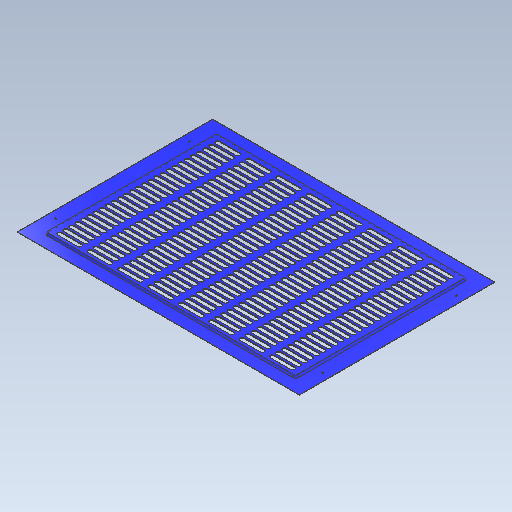
# Autodesk Inventor part: tapa_caja_calor
Saved by Autodesk Inventor 2021 (Build 250183000, 183)
## iProperties
Created: 2021-04-15
Part Number: tapa_caja_calor
Material: Acero AISI 1006 85 LC
Document SubType Name: Chapa
Designer: Leonardo Fabio Mercado Benítez
Density: 7.872 g/cm^3
Sheet Metal Rule: Por defecto_mm
Appearance: Acero
Mass: 732.482 g
Surface Area: 2149.19 cm^2
Volume: 93.049 cm^3
Flat Pattern Width: 32.15 cm
Flat Pattern Length: 46.42 cm
Flat Pattern Area: 1492.4 cm^2
Sheet Metal Width: 321,500 mm
Sheet Metal Length: 464,200 mm
Sheet Metal Area: 149240,300 mm^2
Author: Leonardo Fabio Mercado Benítez
Autodesk Inventor part; units mm, degrees
(part 1 of 3)
ref_plane "YZ Plane" through (0, 0, 0) normal (1, 0, 0) x (0, 1, 0)
ref_plane "XZ Plane" through (0, 0, 0) normal (0, 1, 0) x (-1, 0, 0)
ref_plane "XY Plane" through (0, 0, 0) normal (0, 0, 1) x (1, 0, 0)
sketch "Boceto1" plane through (0, 0, 0) normal (0, 1, 0) x (-1, 0, 0)
  line L0 (232.1, 160.75) -> (-232.1, 160.75)
  line L1 (-232.1, 160.75) -> (-232.1, -160.75)
  line L2 (-232.1, -160.75) -> (232.1, -160.75)
  line L3 (232.1, -160.75) -> (232.1, 160.75)
  line L4 (232.1, 160.75) -> (-232.1, -160.75) construction
  line L5 (-232.1, 160.75) -> (232.1, -160.75) construction
  point P0 (0, 0)
  dimension "d0" = 464.2
  dimension "d1" = 321.5
  measures "d0" distance of L2.end L1.end
  measures "d1" distance of L1.end L0.end
extrude "Placa1" add sketch "Boceto1" along normal blind 0.45
sketch "Boceto3" plane through (0, 0.45, 0) normal (0, 1, 0) x (1, 0, 0)
  line L0 (-201.7, -141.7) -> (201.7, -141.7)
  line L1 (206.7, -136.7) -> (206.7, 136.7)
  line L2 (201.7, 141.7) -> (-201.7, 141.7)
  line L3 (-206.7, 136.7) -> (-206.7, -136.7)
  line L4 (-206.7, -141.7) -> (206.7, 141.7) construction
  line L5 (206.7, -141.7) -> (-206.7, 141.7) construction
  arc A0 (-201.7, 141.7) -> (-206.7, 136.7) centre (-201.7, 136.7) ccw
  arc A1 (206.7, 136.7) -> (201.7, 141.7) centre (201.7, 136.7) ccw
  arc A2 (201.7, -141.7) -> (206.7, -136.7) centre (201.7, -136.7) ccw
  arc A3 (-206.7, -136.7) -> (-201.7, -141.7) centre (-201.7, -136.7) ccw
  line L6 (-201.7, 140.94) -> (201.7, 140.94)
  arc A4 (205.94, 136.7) -> (201.7, 140.94) centre (201.7, 136.7) ccw
  line L7 (205.94, 136.7) -> (205.94, -136.7)
  arc A5 (201.7, -140.94) -> (205.94, -136.7) centre (201.7, -136.7) ccw
  line L8 (201.7, -140.94) -> (-201.7, -140.94)
  arc A6 (-205.94, -136.7) -> (-201.7, -140.94) centre (-201.7, -136.7) ccw
  line L9 (-205.94, -136.7) -> (-205.94, 136.7)
  arc A7 (-201.7, 140.94) -> (-205.94, 136.7) centre (-201.7, 136.7) ccw
  point P0 (0, 0)
  dimension "d3" = 413.4
  dimension "d4" = 283.4
  dimension "d5" = 5
  dimension "d6" = 5
  dimension "d7" = 0.76
  constraints: 20 end point, 16 point on circle, 8 centre point, 8 point on line, 8 tangent, 4 parallel, 2 equal radius, 2 midpoint, 2 perpendicular, 1 horizontal, 7 other
  measures "d3" distance of L5.end L4.end
  measures "d4" distance of L4.end L5.start
  measures "d5" radius of A0
  measures "d6" radius of A1
  measures "d7" distance between parallel lines of L2 L6
sketch "Boceto3 outline for Extrusión1" plane through (0, 0.45, 0) normal (0, 1, 0) x (1, 0, 0)
  line L0 (-201.7, -141.7) -> (201.7, -141.7)
  arc A0 (-206.7, -136.7) -> (-201.7, -141.7) centre (-201.7, -136.7) ccw
  line L1 (-206.7, 136.7) -> (-206.7, -136.7)
  arc A1 (-201.7, 141.7) -> (-206.7, 136.7) centre (-201.7, 136.7) ccw
  line L2 (201.7, 141.7) -> (-201.7, 141.7)
  arc A2 (206.7, 136.7) -> (201.7, 141.7) centre (201.7, 136.7) ccw
  line L3 (206.7, -136.7) -> (206.7, 136.7)
  arc A3 (201.7, -141.7) -> (206.7, -136.7) centre (201.7, -136.7) ccw
extrude "Extrusión1" add sketch "Boceto3 outline for Extrusión1" along normal blind 3.175 draft -30
sketch "Boceto4" plane through (0, 0, 0) normal (0, -1, 0) x (1, 0, 0)
  line L0 (204.866913, -136.7) -> (204.866913, 136.7)
  line L1 (201.7, 139.866913) -> (-201.7, 139.866913)
  arc A0 (204.866913, 136.7) -> (201.7, 139.866913) centre (201.7, 136.7) ccw
  arc A1 (201.7, -139.866913) -> (204.866913, -136.7) centre (201.7, -136.7) ccw
  line L2 (-201.7, -139.866913) -> (201.7, -139.866913)
  arc A2 (-201.7, 139.866913) -> (-204.866913, 136.7) centre (-201.7, 136.7) ccw
  line L3 (-204.866913, 136.7) -> (-204.866913, -136.7)
  arc A3 (-204.866913, -136.7) -> (-201.7, -139.866913) centre (-201.7, -136.7) ccw
  point P0 (0, 0)
extrude "Extrusión2" cut sketch "Boceto4" against normal blind 2.415 draft -30
sketch "Boceto6" plane through (0, 2.415, 0) normal (0, -1, 0) x (1, 0, 0)
  line L0 (-194.972612, 131.472612) -> (-154.972612, 131.472612) construction
  line L1 (-191.622612, 128.122612) -> (-158.322612, 128.122612)
  line L2 (-158.322612, 134.822612) -> (-191.622612, 134.822612)
  arc A0 (-191.622612, 134.822612) -> (-191.622612, 128.122612) centre (-191.622612, 131.472612) ccw
  arc A1 (-158.322612, 128.122612) -> (-158.322612, 134.822612) centre (-158.322612, 131.472612) ccw
  line L3 (-203.472612, 136.7) -> (-203.472612, -136.7)
  line L4 (201.7, 138.472612) -> (-201.7, 138.472612)
  line L5 (-144.972612, 131.472612) -> (-104.972612, 131.472612) construction
  line L6 (-141.622612, 128.122612) -> (-108.322612, 128.122612)
  line L7 (-108.322612, 134.822612) -> (-141.622612, 134.822612)
  arc A2 (-141.622612, 134.822612) -> (-141.622612, 128.122612) centre (-141.622612, 131.472612) ccw
  arc A3 (-108.322612, 128.122612) -> (-108.322612, 134.822612) centre (-108.322612, 131.472612) ccw
  line L8 (-94.972612, 131.472612) -> (-54.972612, 131.472612) construction
  line L9 (-91.622612, 128.122612) -> (-58.322612, 128.122612)
  line L10 (-58.322612, 134.822612) -> (-91.622612, 134.822612)
  arc A4 (-91.622612, 134.822612) -> (-91.622612, 128.122612) centre (-91.622612, 131.472612) ccw
  arc A5 (-58.322612, 128.122612) -> (-58.322612, 134.822612) centre (-58.322612, 131.472612) ccw
  line L11 (-44.972612, 131.472612) -> (-4.972612, 131.472612) construction
  line L12 (-41.622612, 128.122612) -> (-8.322612, 128.122612)
  line L13 (-8.322612, 134.822612) -> (-41.622612, 134.822612)
  arc A6 (-41.622612, 134.822612) -> (-41.622612, 128.122612) centre (-41.622612, 131.472612) ccw
  arc A7 (-8.322612, 128.122612) -> (-8.322612, 134.822612) centre (-8.322612, 131.472612) ccw
  line L14 (5.027388, 131.472612) -> (45.027388, 131.472612) construction
  line L15 (8.377388, 128.122612) -> (41.677388, 128.122612)
  line L16 (41.677388, 134.822612) -> (8.377388, 134.822612)
  arc A8 (8.377388, 134.822612) -> (8.377388, 128.122612) centre (8.377388, 131.472612) ccw
  arc A9 (41.677388, 128.122612) -> (41.677388, 134.822612) centre (41.677388, 131.472612) ccw
  line L17 (55.027388, 131.472612) -> (95.027388, 131.472612) construction
  line L18 (58.377388, 128.122612) -> (91.677388, 128.122612)
  line L19 (91.677388, 134.822612) -> (58.377388, 134.822612)
  arc A10 (58.377388, 134.822612) -> (58.377388, 128.122612) centre (58.377388, 131.472612) ccw
  arc A11 (91.677388, 128.122612) -> (91.677388, 134.822612) centre (91.677388, 131.472612) ccw
  line L20 (105.027388, 131.472612) -> (145.027388, 131.472612) construction
  line L21 (108.377388, 128.122612) -> (141.677388, 128.122612)
  line L22 (141.677388, 134.822612) -> (108.377388, 134.822612)
  arc A12 (108.377388, 134.822612) -> (108.377388, 128.122612) centre (108.377388, 131.472612) ccw
  arc A13 (141.677388, 128.122612) -> (141.677388, 134.822612) centre (141.677388, 131.472612) ccw
  line L23 (155.027388, 131.472612) -> (195.027388, 131.472612) construction
  line L24 (158.377388, 128.122612) -> (191.677388, 128.122612)
  line L25 (191.677388, 134.822612) -> (158.377388, 134.822612)
  arc A14 (158.377388, 134.822612) -> (158.377388, 128.122612) centre (158.377388, 131.472612) ccw
  arc A15 (191.677388, 128.122612) -> (191.677388, 134.822612) centre (191.677388, 131.472612) ccw
  arc A16 (-158.322612, 118.122612) -> (-158.322612, 124.822612) centre (-158.322612, 121.472612) ccw
  line L26 (-191.622612, 118.122612) -> (-158.322612, 118.122612)
  line L27 (-158.322612, 124.822612) -> (-191.622612, 124.822612)
  arc A17 (-191.622612, 124.822612) -> (-191.622612, 118.122612) centre (-191.622612, 121.472612) ccw
  line L28 (-194.972612, 121.472612) -> (-154.972612, 121.472612) construction
  arc A18 (-158.322612, 108.122612) -> (-158.322612, 114.822612) centre (-158.322612, 111.472612) ccw
  line L29 (-191.622612, 108.122612) -> (-158.322612, 108.122612)
  line L30 (-158.322612, 114.822612) -> (-191.622612, 114.822612)
  arc A19 (-191.622612, 114.822612) -> (-191.622612, 108.122612) centre (-191.622612, 111.472612) ccw
  line L31 (-194.972612, 111.472612) -> (-154.972612, 111.472612) construction
  arc A20 (-158.322612, 98.122612) -> (-158.322612, 104.822612) centre (-158.322612, 101.472612) ccw
  line L32 (-191.622612, 98.122612) -> (-158.322612, 98.122612)
  line L33 (-158.322612, 104.822612) -> (-191.622612, 104.822612)
  arc A21 (-191.622612, 104.822612) -> (-191.622612, 98.122612) centre (-191.622612, 101.472612) ccw
  line L34 (-194.972612, 101.472612) -> (-154.972612, 101.472612) construction
  arc A22 (-158.322612, 88.122612) -> (-158.322612, 94.822612) centre (-158.322612, 91.472612) ccw
  line L35 (-191.622612, 88.122612) -> (-158.322612, 88.122612)
  line L36 (-158.322612, 94.822612) -> (-191.622612, 94.822612)
  arc A23 (-191.622612, 94.822612) -> (-191.622612, 88.122612) centre (-191.622612, 91.472612) ccw
  line L37 (-194.972612, 91.472612) -> (-154.972612, 91.472612) construction
  arc A24 (-158.322612, 78.122612) -> (-158.322612, 84.822612) centre (-158.322612, 81.472612) ccw
  line L38 (-191.622612, 78.122612) -> (-158.322612, 78.122612)
  line L39 (-158.322612, 84.822612) -> (-191.622612, 84.822612)
  arc A25 (-191.622612, 84.822612) -> (-191.622612, 78.122612) centre (-191.622612, 81.472612) ccw
  line L40 (-194.972612, 81.472612) -> (-154.972612, 81.472612) construction
  arc A26 (-158.322612, 68.122612) -> (-158.322612, 74.822612) centre (-158.322612, 71.472612) ccw
  line L41 (-191.622612, 68.122612) -> (-158.322612, 68.122612)
  line L42 (-158.322612, 74.822612) -> (-191.622612, 74.822612)
  arc A27 (-191.622612, 74.822612) -> (-191.622612, 68.122612) centre (-191.622612, 71.472612) ccw
  line L43 (-194.972612, 71.472612) -> (-154.972612, 71.472612) construction
  arc A28 (-158.322612, 58.122612) -> (-158.322612, 64.822612) centre (-158.322612, 61.472612) ccw
  line L44 (-191.622612, 58.122612) -> (-158.322612, 58.122612)
  line L45 (-158.322612, 64.822612) -> (-191.622612, 64.822612)
  arc A29 (-191.622612, 64.822612) -> (-191.622612, 58.122612) centre (-191.622612, 61.472612) ccw
  line L46 (-194.972612, 61.472612) -> (-154.972612, 61.472612) construction
  arc A30 (-158.322612, 48.122612) -> (-158.322612, 54.822612) centre (-158.322612, 51.472612) ccw
  line L47 (-191.622612, 48.122612) -> (-158.322612, 48.122612)
  line L48 (-158.322612, 54.822612) -> (-191.622612, 54.822612)
  arc A31 (-191.622612, 54.822612) -> (-191.622612, 48.122612) centre (-191.622612, 51.472612) ccw
  line L49 (-194.972612, 51.472612) -> (-154.972612, 51.472612) construction
  arc A32 (-158.322612, 38.122612) -> (-158.322612, 44.822612) centre (-158.322612, 41.472612) ccw
  line L50 (-191.622612, 38.122612) -> (-158.322612, 38.122612)
  line L51 (-158.322612, 44.822612) -> (-191.622612, 44.822612)
  arc A33 (-191.622612, 44.822612) -> (-191.622612, 38.122612) centre (-191.622612, 41.472612) ccw
  line L52 (-194.972612, 41.472612) -> (-154.972612, 41.472612) construction
  arc A34 (-158.322612, 28.122612) -> (-158.322612, 34.822612) centre (-158.322612, 31.472612) ccw
  line L53 (-191.622612, 28.122612) -> (-158.322612, 28.122612)
  line L54 (-158.322612, 34.822612) -> (-191.622612, 34.822612)
  arc A35 (-191.622612, 34.822612) -> (-191.622612, 28.122612) centre (-191.622612, 31.472612) ccw
  line L55 (-194.972612, 31.472612) -> (-154.972612, 31.472612) construction
  arc A36 (-158.322612, 18.122612) -> (-158.322612, 24.822612) centre (-158.322612, 21.472612) ccw
  line L56 (-191.622612, 18.122612) -> (-158.322612, 18.122612)
  line L57 (-158.322612, 24.822612) -> (-191.622612, 24.822612)
  arc A37 (-191.622612, 24.822612) -> (-191.622612, 18.122612) centre (-191.622612, 21.472612) ccw
  line L58 (-194.972612, 21.472612) -> (-154.972612, 21.472612) construction
  arc A38 (-158.322612, 8.122612) -> (-158.322612, 14.822612) centre (-158.322612, 11.472612) ccw
  line L59 (-191.622612, 8.122612) -> (-158.322612, 8.122612)
  line L60 (-158.322612, 14.822612) -> (-191.622612, 14.822612)
  arc A39 (-191.622612, 14.822612) -> (-191.622612, 8.122612) centre (-191.622612, 11.472612) ccw
  line L61 (-194.972612, 11.472612) -> (-154.972612, 11.472612) construction
  arc A40 (-158.322612, -1.877388) -> (-158.322612, 4.822612) centre (-158.322612, 1.472612) ccw
  line L62 (-191.622612, -1.877388) -> (-158.322612, -1.877388)
  line L63 (-158.322612, 4.822612) -> (-191.622612, 4.822612)
  arc A41 (-191.622612, 4.822612) -> (-191.622612, -1.877388) centre (-191.622612, 1.472612) ccw
  line L64 (-194.972612, 1.472612) -> (-154.972612, 1.472612) construction
  arc A42 (-158.322612, -11.877388) -> (-158.322612, -5.177388) centre (-158.322612, -8.527388) ccw
  line L65 (-191.622612, -11.877388) -> (-158.322612, -11.877388)
  line L66 (-158.322612, -5.177388) -> (-191.622612, -5.177388)
  arc A43 (-191.622612, -5.177388) -> (-191.622612, -11.877388) centre (-191.622612, -8.527388) ccw
  line L67 (-194.972612, -8.527388) -> (-154.972612, -8.527388) construction
  arc A44 (-158.322612, -21.877388) -> (-158.322612, -15.177388) centre (-158.322612, -18.527388) ccw
  line L68 (-191.622612, -21.877388) -> (-158.322612, -21.877388)
  line L69 (-158.322612, -15.177388) -> (-191.622612, -15.177388)
  arc A45 (-191.622612, -15.177388) -> (-191.622612, -21.877388) centre (-191.622612, -18.527388) ccw
  line L70 (-194.972612, -18.527388) -> (-154.972612, -18.527388) construction
  arc A46 (-158.322612, -31.877388) -> (-158.322612, -25.177388) centre (-158.322612, -28.527388) ccw
  line L71 (-191.622612, -31.877388) -> (-158.322612, -31.877388)
  line L72 (-158.322612, -25.177388) -> (-191.622612, -25.177388)
  arc A47 (-191.622612, -25.177388) -> (-191.622612, -31.877388) centre (-191.622612, -28.527388) ccw
  line L73 (-194.972612, -28.527388) -> (-154.972612, -28.527388) construction
  arc A48 (-158.322612, -41.877388) -> (-158.322612, -35.177388) centre (-158.322612, -38.527388) ccw
  line L74 (-191.622612, -41.877388) -> (-158.322612, -41.877388)
  line L75 (-158.322612, -35.177388) -> (-191.622612, -35.177388)
  arc A49 (-191.622612, -35.177388) -> (-191.622612, -41.877388) centre (-191.622612, -38.527388) ccw
  line L76 (-194.972612, -38.527388) -> (-154.972612, -38.527388) construction
  arc A50 (-158.322612, -51.877388) -> (-158.322612, -45.177388) centre (-158.322612, -48.527388) ccw
  line L77 (-191.622612, -51.877388) -> (-158.322612, -51.877388)
  line L78 (-158.322612, -45.177388) -> (-191.622612, -45.177388)
  arc A51 (-191.622612, -45.177388) -> (-191.622612, -51.877388) centre (-191.622612, -48.527388) ccw
  line L79 (-194.972612, -48.527388) -> (-154.972612, -48.527388) construction
  arc A52 (-158.322612, -61.877388) -> (-158.322612, -55.177388) centre (-158.322612, -58.527388) ccw
  line L80 (-191.622612, -61.877388) -> (-158.322612, -61.877388)
  line L81 (-158.322612, -55.177388) -> (-191.622612, -55.177388)
  arc A53 (-191.622612, -55.177388) -> (-191.622612, -61.877388) centre (-191.622612, -58.527388) ccw
  line L82 (-194.972612, -58.527388) -> (-154.972612, -58.527388) construction
  arc A54 (-158.322612, -71.877388) -> (-158.322612, -65.177388) centre (-158.322612, -68.527388) ccw
  line L83 (-191.622612, -71.877388) -> (-158.322612, -71.877388)
  line L84 (-158.322612, -65.177388) -> (-191.622612, -65.177388)
  arc A55 (-191.622612, -65.177388) -> (-191.622612, -71.877388) centre (-191.622612, -68.527388) ccw
  line L85 (-194.972612, -68.527388) -> (-154.972612, -68.527388) construction
  arc A56 (-158.322612, -81.877388) -> (-158.322612, -75.177388) centre (-158.322612, -78.527388) ccw
  line L86 (-191.622612, -81.877388) -> (-158.322612, -81.877388)
  line L87 (-158.322612, -75.177388) -> (-191.622612, -75.177388)
  arc A57 (-191.622612, -75.177388) -> (-191.622612, -81.877388) centre (-191.622612, -78.527388) ccw
  line L88 (-194.972612, -78.527388) -> (-154.972612, -78.527388) construction
  arc A58 (-158.322612, -91.877388) -> (-158.322612, -85.177388) centre (-158.322612, -88.527388) ccw
  line L89 (-191.622612, -91.877388) -> (-158.322612, -91.877388)
  line L90 (-158.322612, -85.177388) -> (-191.622612, -85.177388)
  arc A59 (-191.622612, -85.177388) -> (-191.622612, -91.877388) centre (-191.622612, -88.527388) ccw
  line L91 (-194.972612, -88.527388) -> (-154.972612, -88.527388) construction
  arc A60 (-158.322612, -101.877388) -> (-158.322612, -95.177388) centre (-158.322612, -98.527388) ccw
  line L92 (-191.622612, -101.877388) -> (-158.322612, -101.877388)
  line L93 (-158.322612, -95.177388) -> (-191.622612, -95.177388)
  arc A61 (-191.622612, -95.177388) -> (-191.622612, -101.877388) centre (-191.622612, -98.527388) ccw
  line L94 (-194.972612, -98.527388) -> (-154.972612, -98.527388) construction
  arc A62 (-158.322612, -111.877388) -> (-158.322612, -105.177388) centre (-158.322612, -108.527388) ccw
  line L95 (-191.622612, -111.877388) -> (-158.322612, -111.877388)
  line L96 (-158.322612, -105.177388) -> (-191.622612, -105.177388)
  arc A63 (-191.622612, -105.177388) -> (-191.622612, -111.877388) centre (-191.622612, -108.527388) ccw
  line L97 (-194.972612, -108.527388) -> (-154.972612, -108.527388) construction
  arc A64 (-158.322612, -121.877388) -> (-158.322612, -115.177388) centre (-158.322612, -118.527388) ccw
  line L98 (-191.622612, -121.877388) -> (-158.322612, -121.877388)
  line L99 (-158.322612, -115.177388) -> (-191.622612, -115.177388)
  arc A65 (-191.622612, -115.177388) -> (-191.622612, -121.877388) centre (-191.622612, -118.527388) ccw
  line L100 (-194.972612, -118.527388) -> (-154.972612, -118.527388) construction
  arc A66 (-158.322612, -131.877388) -> (-158.322612, -125.177388) centre (-158.322612, -128.527388) ccw
  line L101 (-191.622612, -131.877388) -> (-158.322612, -131.877388)
  line L102 (-158.322612, -125.177388) -> (-191.622612, -125.177388)
  arc A67 (-191.622612, -125.177388) -> (-191.622612, -131.877388) centre (-191.622612, -128.527388) ccw
  line L103 (-194.972612, -128.527388) -> (-154.972612, -128.527388) construction
  arc A68 (-108.322612, 118.122612) -> (-108.322612, 124.822612) centre (-108.322612, 121.472612) ccw
  line L104 (-141.622612, 118.122612) -> (-108.322612, 118.122612)
  line L105 (-108.322612, 124.822612) -> (-141.622612, 124.822612)
  line L106 (-144.972612, 121.472612) -> (-104.972612, 121.472612) construction
  arc A69 (-141.622612, 124.822612) -> (-141.622612, 118.122612) centre (-141.622612, 121.472612) ccw
  arc A70 (-108.322612, 108.122612) -> (-108.322612, 114.822612) centre (-108.322612, 111.472612) ccw
  line L107 (-141.622612, 108.122612) -> (-108.322612, 108.122612)
  line L108 (-108.322612, 114.822612) -> (-141.622612, 114.822612)
  line L109 (-144.972612, 111.472612) -> (-104.972612, 111.472612) construction
  arc A71 (-141.622612, 114.822612) -> (-141.622612, 108.122612) centre (-141.622612, 111.472612) ccw
  arc A72 (-108.322612, 98.122612) -> (-108.322612, 104.822612) centre (-108.322612, 101.472612) ccw
  line L110 (-141.622612, 98.122612) -> (-108.322612, 98.122612)
  line L111 (-108.322612, 104.822612) -> (-141.622612, 104.822612)
  line L112 (-144.972612, 101.472612) -> (-104.972612, 101.472612) construction
  arc A73 (-141.622612, 104.822612) -> (-141.622612, 98.122612) centre (-141.622612, 101.472612) ccw
  arc A74 (-108.322612, 88.122612) -> (-108.322612, 94.822612) centre (-108.322612, 91.472612) ccw
  line L113 (-141.622612, 88.122612) -> (-108.322612, 88.122612)
  line L114 (-108.322612, 94.822612) -> (-141.622612, 94.822612)
  line L115 (-144.972612, 91.472612) -> (-104.972612, 91.472612) construction
  arc A75 (-141.622612, 94.822612) -> (-141.622612, 88.122612) centre (-141.622612, 91.472612) ccw
  arc A76 (-108.322612, 78.122612) -> (-108.322612, 84.822612) centre (-108.322612, 81.472612) ccw
  line L116 (-141.622612, 78.122612) -> (-108.322612, 78.122612)
  line L117 (-108.322612, 84.822612) -> (-141.622612, 84.822612)
  line L118 (-144.972612, 81.472612) -> (-104.972612, 81.472612) construction
  arc A77 (-141.622612, 84.822612) -> (-141.622612, 78.122612) centre (-141.622612, 81.472612) ccw
  arc A78 (-108.322612, 68.122612) -> (-108.322612, 74.822612) centre (-108.322612, 71.472612) ccw
  line L119 (-141.622612, 68.122612) -> (-108.322612, 68.122612)
  line L120 (-108.322612, 74.822612) -> (-141.622612, 74.822612)
  line L121 (-144.972612, 71.472612) -> (-104.972612, 71.472612) construction
  arc A79 (-141.622612, 74.822612) -> (-141.622612, 68.122612) centre (-141.622612, 71.472612) ccw
  arc A80 (-108.322612, 58.122612) -> (-108.322612, 64.822612) centre (-108.322612, 61.472612) ccw
  line L122 (-141.622612, 58.122612) -> (-108.322612, 58.122612)
  line L123 (-108.322612, 64.822612) -> (-141.622612, 64.822612)
  line L124 (-144.972612, 61.472612) -> (-104.972612, 61.472612) construction
  arc A81 (-141.622612, 64.822612) -> (-141.622612, 58.122612) centre (-141.622612, 61.472612) ccw
  arc A82 (-108.322612, 48.122612) -> (-108.322612, 54.822612) centre (-108.322612, 51.472612) ccw
  line L125 (-141.622612, 48.122612) -> (-108.322612, 48.122612)
  line L126 (-108.322612, 54.822612) -> (-141.622612, 54.822612)
  line L127 (-144.972612, 51.472612) -> (-104.972612, 51.472612) construction
  arc A83 (-141.622612, 54.822612) -> (-141.622612, 48.122612) centre (-141.622612, 51.472612) ccw
  arc A84 (-108.322612, 38.122612) -> (-108.322612, 44.822612) centre (-108.322612, 41.472612) ccw
  line L128 (-141.622612, 38.122612) -> (-108.322612, 38.122612)
  line L129 (-108.322612, 44.822612) -> (-141.622612, 44.822612)
  line L130 (-144.972612, 41.472612) -> (-104.972612, 41.472612) construction
  arc A85 (-141.622612, 44.822612) -> (-141.622612, 38.122612) centre (-141.622612, 41.472612) ccw
  arc A86 (-108.322612, 28.122612) -> (-108.322612, 34.822612) centre (-108.322612, 31.472612) ccw
  line L131 (-141.622612, 28.122612) -> (-108.322612, 28.122612)
  line L132 (-108.322612, 34.822612) -> (-141.622612, 34.822612)
  line L133 (-144.972612, 31.472612) -> (-104.972612, 31.472612) construction
  arc A87 (-141.622612, 34.822612) -> (-141.622612, 28.122612) centre (-141.622612, 31.472612) ccw
  arc A88 (-108.322612, 18.122612) -> (-108.322612, 24.822612) centre (-108.322612, 21.472612) ccw
  line L134 (-141.622612, 18.122612) -> (-108.322612, 18.122612)
  line L135 (-108.322612, 24.822612) -> (-141.622612, 24.822612)
  line L136 (-144.972612, 21.472612) -> (-104.972612, 21.472612) construction
  arc A89 (-141.622612, 24.822612) -> (-141.622612, 18.122612) centre (-141.622612, 21.472612) ccw
  arc A90 (-108.322612, 8.122612) -> (-108.322612, 14.822612) centre (-108.322612, 11.472612) ccw
  line L137 (-141.622612, 8.122612) -> (-108.322612, 8.122612)
  line L138 (-108.322612, 14.822612) -> (-141.622612, 14.822612)
  line L139 (-144.972612, 11.472612) -> (-104.972612, 11.472612) construction
  arc A91 (-141.622612, 14.822612) -> (-141.622612, 8.122612) centre (-141.622612, 11.472612) ccw
  arc A92 (-108.322612, -1.877388) -> (-108.322612, 4.822612) centre (-108.322612, 1.472612) ccw
  line L140 (-141.622612, -1.877388) -> (-108.322612, -1.877388)
  line L141 (-108.322612, 4.822612) -> (-141.622612, 4.822612)
  line L142 (-144.972612, 1.472612) -> (-104.972612, 1.472612) construction
  arc A93 (-141.622612, 4.822612) -> (-141.622612, -1.877388) centre (-141.622612, 1.472612) ccw
  arc A94 (-108.322612, -11.877388) -> (-108.322612, -5.177388) centre (-108.322612, -8.527388) ccw
  line L143 (-141.622612, -11.877388) -> (-108.322612, -11.877388)
  line L144 (-108.322612, -5.177388) -> (-141.622612, -5.177388)
  line L145 (-144.972612, -8.527388) -> (-104.972612, -8.527388) construction
  arc A95 (-141.622612, -5.177388) -> (-141.622612, -11.877388) centre (-141.622612, -8.527388) ccw
  arc A96 (-108.322612, -21.877388) -> (-108.322612, -15.177388) centre (-108.322612, -18.527388) ccw
  line L146 (-141.622612, -21.877388) -> (-108.322612, -21.877388)
  line L147 (-108.322612, -15.177388) -> (-141.622612, -15.177388)
  line L148 (-144.972612, -18.527388) -> (-104.972612, -18.527388) construction
  arc A97 (-141.622612, -15.177388) -> (-141.622612, -21.877388) centre (-141.622612, -18.527388) ccw
  arc A98 (-108.322612, -31.877388) -> (-108.322612, -25.177388) centre (-108.322612, -28.527388) ccw
  line L149 (-141.622612, -31.877388) -> (-108.322612, -31.877388)
  line L150 (-108.322612, -25.177388) -> (-141.622612, -25.177388)
  line L151 (-144.972612, -28.527388) -> (-104.972612, -28.527388) construction
  arc A99 (-141.622612, -25.177388) -> (-141.622612, -31.877388) centre (-141.622612, -28.527388) ccw
  arc A100 (-108.322612, -41.877388) -> (-108.322612, -35.177388) centre (-108.322612, -38.527388) ccw
  line L152 (-141.622612, -41.877388) -> (-108.322612, -41.877388)
  line L153 (-108.322612, -35.177388) -> (-141.622612, -35.177388)
  line L154 (-144.972612, -38.527388) -> (-104.972612, -38.527388) construction
  arc A101 (-141.622612, -35.177388) -> (-141.622612, -41.877388) centre (-141.622612, -38.527388) ccw
  arc A102 (-108.322612, -51.877388) -> (-108.322612, -45.177388) centre (-108.322612, -48.527388) ccw
  line L155 (-141.622612, -51.877388) -> (-108.322612, -51.877388)
  line L156 (-108.322612, -45.177388) -> (-141.622612, -45.177388)
  line L157 (-144.972612, -48.527388) -> (-104.972612, -48.527388) construction
  arc A103 (-141.622612, -45.177388) -> (-141.622612, -51.877388) centre (-141.622612, -48.527388) ccw
  arc A104 (-108.322612, -61.877388) -> (-108.322612, -55.177388) centre (-108.322612, -58.527388) ccw
  line L158 (-141.622612, -61.877388) -> (-108.322612, -61.877388)
  line L159 (-108.322612, -55.177388) -> (-141.622612, -55.177388)
  line L160 (-144.972612, -58.527388) -> (-104.972612, -58.527388) construction
  arc A105 (-141.622612, -55.177388) -> (-141.622612, -61.877388) centre (-141.622612, -58.527388) ccw
  arc A106 (-108.322612, -71.877388) -> (-108.322612, -65.177388) centre (-108.322612, -68.527388) ccw
  line L161 (-141.622612, -71.877388) -> (-108.322612, -71.877388)
  line L162 (-108.322612, -65.177388) -> (-141.622612, -65.177388)
  line L163 (-144.972612, -68.527388) -> (-104.972612, -68.527388) construction
  arc A107 (-141.622612, -65.177388) -> (-141.622612, -71.877388) centre (-141.622612, -68.527388) ccw
  arc A108 (-108.322612, -81.877388) -> (-108.322612, -75.177388) centre (-108.322612, -78.527388) ccw
  line L164 (-141.622612, -81.877388) -> (-108.322612, -81.877388)
  line L165 (-108.322612, -75.177388) -> (-141.622612, -75.177388)
  line L166 (-144.972612, -78.527388) -> (-104.972612, -78.527388) construction
  arc A109 (-141.622612, -75.177388) -> (-141.622612, -81.877388) centre (-141.622612, -78.527388) ccw
  arc A110 (-108.322612, -91.877388) -> (-108.322612, -85.177388) centre (-108.322612, -88.527388) ccw
  line L167 (-141.622612, -91.877388) -> (-108.322612, -91.877388)
  line L168 (-108.322612, -85.177388) -> (-141.622612, -85.177388)
  line L169 (-144.972612, -88.527388) -> (-104.972612, -88.527388) construction
  arc A111 (-141.622612, -85.177388) -> (-141.622612, -91.877388) centre (-141.622612, -88.527388) ccw
  arc A112 (-108.322612, -101.877388) -> (-108.322612, -95.177388) centre (-108.322612, -98.527388) ccw
  line L170 (-141.622612, -101.877388) -> (-108.322612, -101.877388)
  line L171 (-108.322612, -95.177388) -> (-141.622612, -95.177388)
  line L172 (-144.972612, -98.527388) -> (-104.972612, -98.527388) construction
  arc A113 (-141.622612, -95.177388) -> (-141.622612, -101.877388) centre (-141.622612, -98.527388) ccw
  arc A114 (-108.322612, -111.877388) -> (-108.322612, -105.177388) centre (-108.322612, -108.527388) ccw
  line L173 (-141.622612, -111.877388) -> (-108.322612, -111.877388)
  line L174 (-108.322612, -105.177388) -> (-141.622612, -105.177388)
  line L175 (-144.972612, -108.527388) -> (-104.972612, -108.527388) construction
  arc A115 (-141.622612, -105.177388) -> (-141.622612, -111.877388) centre (-141.622612, -108.527388) ccw
  arc A116 (-108.322612, -121.877388) -> (-108.322612, -115.177388) centre (-108.322612, -118.527388) ccw
  line L176 (-141.622612, -121.877388) -> (-108.322612, -121.877388)
  line L177 (-108.322612, -115.177388) -> (-141.622612, -115.177388)
  line L178 (-144.972612, -118.527388) -> (-104.972612, -118.527388) construction
  arc A117 (-141.622612, -115.177388) -> (-141.622612, -121.877388) centre (-141.622612, -118.527388) ccw
  arc A118 (-108.322612, -131.877388) -> (-108.322612, -125.177388) centre (-108.322612, -128.527388) ccw
  line L179 (-141.622612, -131.877388) -> (-108.322612, -131.877388)
  line L180 (-108.322612, -125.177388) -> (-141.622612, -125.177388)
  line L181 (-144.972612, -128.527388) -> (-104.972612, -128.527388) construction
  arc A119 (-141.622612, -125.177388) -> (-141.622612, -131.877388) centre (-141.622612, -128.527388) ccw
  arc A120 (-41.622612, 124.822612) -> (-41.622612, 118.122612) centre (-41.622612, 121.472612) ccw
  line L182 (-41.622612, 118.122612) -> (-8.322612, 118.122612)
  line L183 (-8.322612, 124.822612) -> (-41.622612, 124.822612)
  line L184 (-44.972612, 121.472612) -> (-4.972612, 121.472612) construction
  arc A121 (-8.322612, 118.122612) -> (-8.322612, 124.822612) centre (-8.322612, 121.472612) ccw
  arc A122 (8.377388, 124.822612) -> (8.377388, 118.122612) centre (8.377388, 121.472612) ccw
  line L185 (8.377388, 118.122612) -> (41.677388, 118.122612)
  line L186 (41.677388, 124.822612) -> (8.377388, 124.822612)
  line L187 (5.027388, 121.472612) -> (45.027388, 121.472612) construction
  arc A123 (58.377388, 124.822612) -> (58.377388, 118.122612) centre (58.377388, 121.472612) ccw
  line L188 (58.377388, 118.122612) -> (91.677388, 118.122612)
  line L189 (91.677388, 124.822612) -> (58.377388, 124.822612)
  line L190 (55.027388, 121.472612) -> (95.027388, 121.472612) construction
  arc A124 (41.677388, 118.122612) -> (41.677388, 124.822612) centre (41.677388, 121.472612) ccw
  arc A125 (158.377388, 124.822612) -> (158.377388, 118.122612) centre (158.377388, 121.472612) ccw
  line L191 (158.377388, 118.122612) -> (191.677388, 118.122612)
  line L192 (191.677388, 124.822612) -> (158.377388, 124.822612)
  line L193 (155.027388, 121.472612) -> (195.027388, 121.472612) construction
  arc A126 (191.677388, 118.122612) -> (191.677388, 124.822612) centre (191.677388, 121.472612) ccw
  arc A127 (141.677388, 118.122612) -> (141.677388, 124.822612) centre (141.677388, 121.472612) ccw
  line L194 (108.377388, 118.122612) -> (141.677388, 118.122612)
  line L195 (141.677388, 124.822612) -> (108.377388, 124.822612)
  line L196 (105.027388, 121.472612) -> (145.027388, 121.472612) construction
  arc A128 (108.377388, 124.822612) -> (108.377388, 118.122612) centre (108.377388, 121.472612) ccw
  arc A129 (91.677388, 118.122612) -> (91.677388, 124.822612) centre (91.677388, 121.472612) ccw
  arc A130 (-58.322612, 118.122612) -> (-58.322612, 124.822612) centre (-58.322612, 121.472612) ccw
  line L197 (-91.622612, 118.122612) -> (-58.322612, 118.122612)
  line L198 (-58.322612, 124.822612) -> (-91.622612, 124.822612)
  line L199 (-94.972612, 121.472612) -> (-54.972612, 121.472612) construction
  arc A131 (-91.622612, 124.822612) -> (-91.622612, 118.122612) centre (-91.622612, 121.472612) ccw
  arc A132 (-41.622612, 114.822612) -> (-41.622612, 108.122612) centre (-41.622612, 111.472612) ccw
  line L200 (-41.622612, 108.122612) -> (-8.322612, 108.122612)
  line L201 (-8.322612, 114.822612) -> (-41.622612, 114.822612)
  line L202 (-44.972612, 111.472612) -> (-4.972612, 111.472612) construction
  arc A133 (-8.322612, 108.122612) -> (-8.322612, 114.822612) centre (-8.322612, 111.472612) ccw
  arc A134 (8.377388, 114.822612) -> (8.377388, 108.122612) centre (8.377388, 111.472612) ccw
  line L203 (8.377388, 108.122612) -> (41.677388, 108.122612)
  line L204 (41.677388, 114.822612) -> (8.377388, 114.822612)
  line L205 (5.027388, 111.472612) -> (45.027388, 111.472612) construction
  arc A135 (58.377388, 114.822612) -> (58.377388, 108.122612) centre (58.377388, 111.472612) ccw
  line L206 (58.377388, 108.122612) -> (91.677388, 108.122612)
  line L207 (91.677388, 114.822612) -> (58.377388, 114.822612)
  line L208 (55.027388, 111.472612) -> (95.027388, 111.472612) construction
  arc A136 (41.677388, 108.122612) -> (41.677388, 114.822612) centre (41.677388, 111.472612) ccw
  arc A137 (158.377388, 114.822612) -> (158.377388, 108.122612) centre (158.377388, 111.472612) ccw
  line L209 (158.377388, 108.122612) -> (191.677388, 108.122612)
  line L210 (191.677388, 114.822612) -> (158.377388, 114.822612)
  line L211 (155.027388, 111.472612) -> (195.027388, 111.472612) construction
  arc A138 (191.677388, 108.122612) -> (191.677388, 114.822612) centre (191.677388, 111.472612) ccw
  arc A139 (141.677388, 108.122612) -> (141.677388, 114.822612) centre (141.677388, 111.472612) ccw
  line L212 (108.377388, 108.122612) -> (141.677388, 108.122612)
  line L213 (141.677388, 114.822612) -> (108.377388, 114.822612)
  line L214 (105.027388, 111.472612) -> (145.027388, 111.472612) construction
  arc A140 (108.377388, 114.822612) -> (108.377388, 108.122612) centre (108.377388, 111.472612) ccw
  arc A141 (91.677388, 108.122612) -> (91.677388, 114.822612) centre (91.677388, 111.472612) ccw
  arc A142 (-58.322612, 108.122612) -> (-58.322612, 114.822612) centre (-58.322612, 111.472612) ccw
  line L215 (-91.622612, 108.122612) -> (-58.322612, 108.122612)
  line L216 (-58.322612, 114.822612) -> (-91.622612, 114.822612)
  line L217 (-94.972612, 111.472612) -> (-54.972612, 111.472612) construction
  arc A143 (-91.622612, 114.822612) -> (-91.622612, 108.122612) centre (-91.622612, 111.472612) ccw
  arc A144 (-41.622612, 104.822612) -> (-41.622612, 98.122612) centre (-41.622612, 101.472612) ccw
  line L218 (-41.622612, 98.122612) -> (-8.322612, 98.122612)
  line L219 (-8.322612, 104.822612) -> (-41.622612, 104.822612)
  line L220 (-44.972612, 101.472612) -> (-4.972612, 101.472612) construction
  arc A145 (-8.322612, 98.122612) -> (-8.322612, 104.822612) centre (-8.322612, 101.472612) ccw
  arc A146 (8.377388, 104.822612) -> (8.377388, 98.122612) centre (8.377388, 101.472612) ccw
  line L221 (8.377388, 98.122612) -> (41.677388, 98.122612)
  line L222 (41.677388, 104.822612) -> (8.377388, 104.822612)
  line L223 (5.027388, 101.472612) -> (45.027388, 101.472612) construction
  arc A147 (58.377388, 104.822612) -> (58.377388, 98.122612) centre (58.377388, 101.472612) ccw
  line L224 (58.377388, 98.122612) -> (91.677388, 98.122612)
  line L225 (91.677388, 104.822612) -> (58.377388, 104.822612)
  line L226 (55.027388, 101.472612) -> (95.027388, 101.472612) construction
  arc A148 (41.677388, 98.122612) -> (41.677388, 104.822612) centre (41.677388, 101.472612) ccw
  arc A149 (158.377388, 104.822612) -> (158.377388, 98.122612) centre (158.377388, 101.472612) ccw
  line L227 (158.377388, 98.122612) -> (191.677388, 98.122612)
  line L228 (191.677388, 104.822612) -> (158.377388, 104.822612)
  line L229 (155.027388, 101.472612) -> (195.027388, 101.472612) construction
  arc A150 (191.677388, 98.122612) -> (191.677388, 104.822612) centre (191.677388, 101.472612) ccw
  arc A151 (141.677388, 98.122612) -> (141.677388, 104.822612) centre (141.677388, 101.472612) ccw
  line L230 (108.377388, 98.122612) -> (141.677388, 98.122612)
  line L231 (141.677388, 104.822612) -> (108.377388, 104.822612)
  line L232 (105.027388, 101.472612) -> (145.027388, 101.472612) construction
  arc A152 (108.377388, 104.822612) -> (108.377388, 98.122612) centre (108.377388, 101.472612) ccw
  arc A153 (91.677388, 98.122612) -> (91.677388, 104.822612) centre (91.677388, 101.472612) ccw
  arc A154 (-58.322612, 98.122612) -> (-58.322612, 104.822612) centre (-58.322612, 101.472612) ccw
  line L233 (-91.622612, 98.122612) -> (-58.322612, 98.122612)
  line L234 (-58.322612, 104.822612) -> (-91.622612, 104.822612)
  line L235 (-94.972612, 101.472612) -> (-54.972612, 101.472612) construction
  arc A155 (-91.622612, 104.822612) -> (-91.622612, 98.122612) centre (-91.622612, 101.472612) ccw
  arc A156 (-41.622612, 94.822612) -> (-41.622612, 88.122612) centre (-41.622612, 91.472612) ccw
  line L236 (-41.622612, 88.122612) -> (-8.322612, 88.122612)
  line L237 (-8.322612, 94.822612) -> (-41.622612, 94.822612)
  line L238 (-44.972612, 91.472612) -> (-4.972612, 91.472612) construction
  arc A157 (-8.322612, 88.122612) -> (-8.322612, 94.822612) centre (-8.322612, 91.472612) ccw
  arc A158 (8.377388, 94.822612) -> (8.377388, 88.122612) centre (8.377388, 91.472612) ccw
  line L239 (8.377388, 88.122612) -> (41.677388, 88.122612)
  line L240 (41.677388, 94.822612) -> (8.377388, 94.822612)
  line L241 (5.027388, 91.472612) -> (45.027388, 91.472612) construction
  arc A159 (58.377388, 94.822612) -> (58.377388, 88.122612) centre (58.377388, 91.472612) ccw
  line L242 (58.377388, 88.122612) -> (91.677388, 88.122612)
  line L243 (91.677388, 94.822612) -> (58.377388, 94.822612)
  line L244 (55.027388, 91.472612) -> (95.027388, 91.472612) construction
  arc A160 (41.677388, 88.122612) -> (41.677388, 94.822612) centre (41.677388, 91.472612) ccw
  arc A161 (158.377388, 94.822612) -> (158.377388, 88.122612) centre (158.377388, 91.472612) ccw
  line L245 (158.377388, 88.122612) -> (191.677388, 88.122612)
  line L246 (191.677388, 94.822612) -> (158.377388, 94.822612)
  line L247 (155.027388, 91.472612) -> (195.027388, 91.472612) construction
  arc A162 (191.677388, 88.122612) -> (191.677388, 94.822612) centre (191.677388, 91.472612) ccw
  arc A163 (141.677388, 88.122612) -> (141.677388, 94.822612) centre (141.677388, 91.472612) ccw
  line L248 (108.377388, 88.122612) -> (141.677388, 88.122612)
  line L249 (141.677388, 94.822612) -> (108.377388, 94.822612)
  line L250 (105.027388, 91.472612) -> (145.027388, 91.472612) construction
  arc A164 (108.377388, 94.822612) -> (108.377388, 88.122612) centre (108.377388, 91.472612) ccw
  arc A165 (91.677388, 88.122612) -> (91.677388, 94.822612) centre (91.677388, 91.472612) ccw
  arc A166 (-58.322612, 88.122612) -> (-58.322612, 94.822612) centre (-58.322612, 91.472612) ccw
  line L251 (-91.622612, 88.122612) -> (-58.322612, 88.122612)
  line L252 (-58.322612, 94.822612) -> (-91.622612, 94.822612)
  line L253 (-94.972612, 91.472612) -> (-54.972612, 91.472612) construction
  arc A167 (-91.622612, 94.822612) -> (-91.622612, 88.122612) centre (-91.622612, 91.472612) ccw
  arc A168 (-41.622612, 84.822612) -> (-41.622612, 78.122612) centre (-41.622612, 81.472612) ccw
  line L254 (-41.622612, 78.122612) -> (-8.322612, 78.122612)
  line L255 (-8.322612, 84.822612) -> (-41.622612, 84.822612)
  line L256 (-44.972612, 81.472612) -> (-4.972612, 81.472612) construction
  arc A169 (-8.322612, 78.122612) -> (-8.322612, 84.822612) centre (-8.322612, 81.472612) ccw
  arc A170 (8.377388, 84.822612) -> (8.377388, 78.122612) centre (8.377388, 81.472612) ccw
  line L257 (8.377388, 78.122612) -> (41.677388, 78.122612)
  line L258 (41.677388, 84.822612) -> (8.377388, 84.822612)
  line L259 (5.027388, 81.472612) -> (45.027388, 81.472612) construction
  arc A171 (58.377388, 84.822612) -> (58.377388, 78.122612) centre (58.377388, 81.472612) ccw
  line L260 (58.377388, 78.122612) -> (91.677388, 78.122612)
  line L261 (91.677388, 84.822612) -> (58.377388, 84.822612)
  line L262 (55.027388, 81.472612) -> (95.027388, 81.472612) construction
  arc A172 (41.677388, 78.122612) -> (41.677388, 84.822612) centre (41.677388, 81.472612) ccw
  arc A173 (158.377388, 84.822612) -> (158.377388, 78.122612) centre (158.377388, 81.472612) ccw
  line L263 (158.377388, 78.122612) -> (191.677388, 78.122612)
  line L264 (191.677388, 84.822612) -> (158.377388, 84.822612)
  line L265 (155.027388, 81.472612) -> (195.027388, 81.472612) construction
  arc A174 (191.677388, 78.122612) -> (191.677388, 84.822612) centre (191.677388, 81.472612) ccw
  arc A175 (141.677388, 78.122612) -> (141.677388, 84.822612) centre (141.677388, 81.472612) ccw
  line L266 (108.377388, 78.122612) -> (141.677388, 78.122612)
  line L267 (141.677388, 84.822612) -> (108.377388, 84.822612)
  line L268 (105.027388, 81.472612) -> (145.027388, 81.472612) construction
  arc A176 (108.377388, 84.822612) -> (108.377388, 78.122612) centre (108.377388, 81.472612) ccw
  arc A177 (91.677388, 78.122612) -> (91.677388, 84.822612) centre (91.677388, 81.472612) ccw
  arc A178 (-58.322612, 78.122612) -> (-58.322612, 84.822612) centre (-58.322612, 81.472612) ccw
  line L269 (-91.622612, 78.122612) -> (-58.322612, 78.122612)
  line L270 (-58.322612, 84.822612) -> (-91.622612, 84.822612)
  line L271 (-94.972612, 81.472612) -> (-54.972612, 81.472612) construction
  arc A179 (-91.622612, 84.822612) -> (-91.622612, 78.122612) centre (-91.622612, 81.472612) ccw
  arc A180 (-41.622612, 74.822612) -> (-41.622612, 68.122612) centre (-41.622612, 71.472612) ccw
  line L272 (-41.622612, 68.122612) -> (-8.322612, 68.122612)
  line L273 (-8.322612, 74.822612) -> (-41.622612, 74.822612)
  line L274 (-44.972612, 71.472612) -> (-4.972612, 71.472612) construction
  arc A181 (-8.322612, 68.122612) -> (-8.322612, 74.822612) centre (-8.322612, 71.472612) ccw
  arc A182 (8.377388, 74.822612) -> (8.377388, 68.122612) centre (8.377388, 71.472612) ccw
  line L275 (8.377388, 68.122612) -> (41.677388, 68.122612)
  line L276 (41.677388, 74.822612) -> (8.377388, 74.822612)
  line L277 (5.027388, 71.472612) -> (45.027388, 71.472612) construction
  arc A183 (58.377388, 74.822612) -> (58.377388, 68.122612) centre (58.377388, 71.472612) ccw
  line L278 (58.377388, 68.122612) -> (91.677388, 68.122612)
  line L279 (91.677388, 74.822612) -> (58.377388, 74.822612)
  line L280 (55.027388, 71.472612) -> (95.027388, 71.472612) construction
  arc A184 (41.677388, 68.122612) -> (41.677388, 74.822612) centre (41.677388, 71.472612) ccw
  arc A185 (158.377388, 74.822612) -> (158.377388, 68.122612) centre (158.377388, 71.472612) ccw
  line L281 (158.377388, 68.122612) -> (191.677388, 68.122612)
  line L282 (191.677388, 74.822612) -> (158.377388, 74.822612)
  line L283 (155.027388, 71.472612) -> (195.027388, 71.472612) construction
  arc A186 (191.677388, 68.122612) -> (191.677388, 74.822612) centre (191.677388, 71.472612) ccw
  arc A187 (141.677388, 68.122612) -> (141.677388, 74.822612) centre (141.677388, 71.472612) ccw
  line L284 (108.377388, 68.122612) -> (141.677388, 68.122612)
  line L285 (141.677388, 74.822612) -> (108.377388, 74.822612)
  line L286 (105.027388, 71.472612) -> (145.027388, 71.472612) construction
  arc A188 (108.377388, 74.822612) -> (108.377388, 68.122612) centre (108.377388, 71.472612) ccw
  arc A189 (91.677388, 68.122612) -> (91.677388, 74.822612) centre (91.677388, 71.472612) ccw
  arc A190 (-58.322612, 68.122612) -> (-58.322612, 74.822612) centre (-58.322612, 71.472612) ccw
  line L287 (-91.622612, 68.122612) -> (-58.322612, 68.122612)
  line L288 (-58.322612, 74.822612) -> (-91.622612, 74.822612)
  line L289 (-94.972612, 71.472612) -> (-54.972612, 71.472612) construction
  arc A191 (-91.622612, 74.822612) -> (-91.622612, 68.122612) centre (-91.622612, 71.472612) ccw
  arc A192 (-41.622612, 64.822612) -> (-41.622612, 58.122612) centre (-41.622612, 61.472612) ccw
  line L290 (-41.622612, 58.122612) -> (-8.322612, 58.122612)
  line L291 (-8.322612, 64.822612) -> (-41.622612, 64.822612)
  line L292 (-44.972612, 61.472612) -> (-4.972612, 61.472612) construction
  arc A193 (-8.322612, 58.122612) -> (-8.322612, 64.822612) centre (-8.322612, 61.472612) ccw
  arc A194 (8.377388, 64.822612) -> (8.377388, 58.122612) centre (8.377388, 61.472612) ccw
  line L293 (8.377388, 58.122612) -> (41.677388, 58.122612)
  line L294 (41.677388, 64.822612) -> (8.377388, 64.822612)
  line L295 (5.027388, 61.472612) -> (45.027388, 61.472612) construction
  arc A195 (58.377388, 64.822612) -> (58.377388, 58.122612) centre (58.377388, 61.472612) ccw
  line L296 (58.377388, 58.122612) -> (91.677388, 58.122612)
  line L297 (91.677388, 64.822612) -> (58.377388, 64.822612)
  line L298 (55.027388, 61.472612) -> (95.027388, 61.472612) construction
  arc A196 (41.677388, 58.122612) -> (41.677388, 64.822612) centre (41.677388, 61.472612) ccw
  arc A197 (158.377388, 64.822612) -> (158.377388, 58.122612) centre (158.377388, 61.472612) ccw
  line L299 (158.377388, 58.122612) -> (191.677388, 58.122612)
  line L300 (191.677388, 64.822612) -> (158.377388, 64.822612)
  line L301 (155.027388, 61.472612) -> (195.027388, 61.472612) construction
  arc A198 (191.677388, 58.122612) -> (191.677388, 64.822612) centre (191.677388, 61.472612) ccw
  arc A199 (141.677388, 58.122612) -> (141.677388, 64.822612) centre (141.677388, 61.472612) ccw
  line L302 (108.377388, 58.122612) -> (141.677388, 58.122612)
  line L303 (141.677388, 64.822612) -> (108.377388, 64.822612)
  line L304 (105.027388, 61.472612) -> (145.027388, 61.472612) construction
  arc A200 (108.377388, 64.822612) -> (108.377388, 58.122612) centre (108.377388, 61.472612) ccw
  arc A201 (91.677388, 58.122612) -> (91.677388, 64.822612) centre (91.677388, 61.472612) ccw
  arc A202 (-58.322612, 58.122612) -> (-58.322612, 64.822612) centre (-58.322612, 61.472612) ccw
  line L305 (-91.622612, 58.122612) -> (-58.322612, 58.122612)
  line L306 (-58.322612, 64.822612) -> (-91.622612, 64.822612)
  line L307 (-94.972612, 61.472612) -> (-54.972612, 61.472612) construction
  arc A203 (-91.622612, 64.822612) -> (-91.622612, 58.122612) centre (-91.622612, 61.472612) ccw
  arc A204 (-41.622612, 54.822612) -> (-41.622612, 48.122612) centre (-41.622612, 51.472612) ccw
  line L308 (-41.622612, 48.122612) -> (-8.322612, 48.122612)
  line L309 (-8.322612, 54.822612) -> (-41.622612, 54.822612)
  line L310 (-44.972612, 51.472612) -> (-4.972612, 51.472612) construction
  arc A205 (-8.322612, 48.122612) -> (-8.322612, 54.822612) centre (-8.322612, 51.472612) ccw
  arc A206 (8.377388, 54.822612) -> (8.377388, 48.122612) centre (8.377388, 51.472612) ccw
  line L311 (8.377388, 48.122612) -> (41.677388, 48.122612)
  line L312 (41.677388, 54.822612) -> (8.377388, 54.822612)
  line L313 (5.027388, 51.472612) -> (45.027388, 51.472612) construction
  arc A207 (58.377388, 54.822612) -> (58.377388, 48.122612) centre (58.377388, 51.472612) ccw
  line L314 (58.377388, 48.122612) -> (91.677388, 48.122612)
  line L315 (91.677388, 54.822612) -> (58.377388, 54.822612)
  line L316 (55.027388, 51.472612) -> (95.027388, 51.472612) construction
  arc A208 (41.677388, 48.122612) -> (41.677388, 54.822612) centre (41.677388, 51.472612) ccw
  arc A209 (158.377388, 54.822612) -> (158.377388, 48.122612) centre (158.377388, 51.472612) ccw
  line L317 (158.377388, 48.122612) -> (191.677388, 48.122612)
  line L318 (191.677388, 54.822612) -> (158.377388, 54.822612)
  line L319 (155.027388, 51.472612) -> (195.027388, 51.472612) construction
  arc A210 (191.677388, 48.122612) -> (191.677388, 54.822612) centre (191.677388, 51.472612) ccw
  arc A211 (141.677388, 48.122612) -> (141.677388, 54.822612) centre (141.677388, 51.472612) ccw
  line L320 (108.377388, 48.122612) -> (141.677388, 48.122612)
  line L321 (141.677388, 54.822612) -> (108.377388, 54.822612)
  line L322 (105.027388, 51.472612) -> (145.027388, 51.472612) construction
  arc A212 (108.377388, 54.822612) -> (108.377388, 48.122612) centre (108.377388, 51.472612) ccw
  arc A213 (91.677388, 48.122612) -> (91.677388, 54.822612) centre (91.677388, 51.472612) ccw
  arc A214 (-58.322612, 48.122612) -> (-58.322612, 54.822612) centre (-58.322612, 51.472612) ccw
  line L323 (-91.622612, 48.122612) -> (-58.322612, 48.122612)
  line L324 (-58.322612, 54.822612) -> (-91.622612, 54.822612)
  line L325 (-94.972612, 51.472612) -> (-54.972612, 51.472612) construction
  arc A215 (-91.622612, 54.822612) -> (-91.622612, 48.122612) centre (-91.622612, 51.472612) ccw
  arc A216 (-41.622612, 44.822612) -> (-41.622612, 38.122612) centre (-41.622612, 41.472612) ccw
  line L326 (-41.622612, 38.122612) -> (-8.322612, 38.122612)
  line L327 (-8.322612, 44.822612) -> (-41.622612, 44.822612)
  line L328 (-44.972612, 41.472612) -> (-4.972612, 41.472612) construction
  arc A217 (-8.322612, 38.122612) -> (-8.322612, 44.822612) centre (-8.322612, 41.472612) ccw
  arc A218 (8.377388, 44.822612) -> (8.377388, 38.122612) centre (8.377388, 41.472612) ccw
  line L329 (8.377388, 38.122612) -> (41.677388, 38.122612)
  line L330 (41.677388, 44.822612) -> (8.377388, 44.822612)
  line L331 (5.027388, 41.472612) -> (45.027388, 41.472612) construction
  arc A219 (58.377388, 44.822612) -> (58.377388, 38.122612) centre (58.377388, 41.472612) ccw
  line L332 (58.377388, 38.122612) -> (91.677388, 38.122612)
  line L333 (91.677388, 44.822612) -> (58.377388, 44.822612)
  line L334 (55.027388, 41.472612) -> (95.027388, 41.472612) construction
  arc A220 (41.677388, 38.122612) -> (41.677388, 44.822612) centre (41.677388, 41.472612) ccw
  arc A221 (158.377388, 44.822612) -> (158.377388, 38.122612) centre (158.377388, 41.472612) ccw
  line L335 (158.377388, 38.122612) -> (191.677388, 38.122612)
  line L336 (191.677388, 44.822612) -> (158.377388, 44.822612)
  line L337 (155.027388, 41.472612) -> (195.027388, 41.472612) construction
  arc A222 (191.677388, 38.122612) -> (191.677388, 44.822612) centre (191.677388, 41.472612) ccw
  arc A223 (141.677388, 38.122612) -> (141.677388, 44.822612) centre (141.677388, 41.472612) ccw
  line L338 (108.377388, 38.122612) -> (141.677388, 38.122612)
  line L339 (141.677388, 44.822612) -> (108.377388, 44.822612)